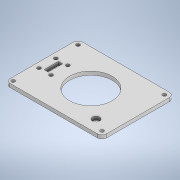
# Autodesk Inventor part: upper_plate_impeller
Saved by Autodesk Inventor 2020 (Build 240168000, 168)
## iProperties
Created: 2023-05-24
Part Number: upper_plate_impeller
Material: Типовые
Document SubType Name: Modeling
Designer: Администратор
Density: 1 g/cm^3
Appearance: По умолчанию
Author: Администратор
Autodesk Inventor part; units mm, degrees
ref_plane "YZ Plane" through (0, 0, 0) normal (1, 0, 0) x (0, 1, 0)
ref_plane "XZ Plane" through (0, 0, 0) normal (0, 1, 0) x (-1, 0, 0)
ref_plane "XY Plane" through (0, 0, 0) normal (0, 0, 1) x (1, 0, 0)
sketch "Эскиз1" plane through (0, 0, 0) normal (0, 1, 0) x (-1, 0, 0)
  line L0 (37, 30) -> (-36, 30)
  line L1 (-40, 26) -> (-40, -26)
  line L2 (-36, -30) -> (36, -30)
  line L3 (40, -26) -> (40, 27)
  line L4 (40, 30) -> (-40, -30) construction
  line L5 (-40, 30) -> (40, -30) construction
  arc A0 (36, -30) -> (40, -26) centre (36, -26) ccw
  arc A1 (40, 27) -> (37, 30) centre (37, 27) ccw
  arc A2 (-40, -26) -> (-36, -30) centre (-36, -26) ccw
  arc A3 (-36, 30) -> (-40, 26) centre (-36, 26) ccw
  circle A4 centre (36, -26) radius 1.5
  circle A5 centre (-36, -26) radius 1.5
  circle A6 centre (-36, 26) radius 1.5
  circle A7 centre (37, 27) radius 1.5
  circle A8 centre (-0.75, 0) radius 17.75
  circle A9 centre (-25, 20) radius 3
  line L6 (40, 0) -> (-40, 0) construction
  circle A10 centre (35.5, -7) radius 1.5
  circle A11 centre (25.5, -7) radius 1.5
  circle A12 centre (35.5, 7) radius 1.5
  circle A13 centre (25.5, 7) radius 1.5
  line L7 (40, 0) -> (23, 0) construction
  line L8 (35.5, -7) -> (25.5, 7) construction
  line L9 (39, -10.5) -> (22, -10.5) construction
  line L10 (22, -10.5) -> (22, 10.5) construction
  line L11 (22, 10.5) -> (39, 10.5) construction
  line L12 (39, 10.5) -> (39, -10.5) construction
  line L13 (32.25, 6) -> (28.75, 6)
  line L14 (28.75, 6) -> (28.75, -6)
  line L15 (28.75, -6) -> (32.25, -6)
  line L16 (32.25, -6) -> (32.25, 6)
  point P0 (0, 0)
  point P1 (30.5, 0)
  dimension "d0" = 80
  dimension "d1" = 60
  dimension "d2" = 4
  dimension "d3" = 3
  dimension "d4" = 4
  dimension "d5" = 3
  dimension "d6" = 3
  dimension "d7" = 3
  dimension "d8" = 3
  dimension "d9" = 35.5
  dimension "d10" = 40.75
  dimension "d13" = 6
  dimension "d14" = 10
  dimension "d15" = 15
  dimension "d16" = 3
  dimension "d17" = 7
  dimension "d18" = 4.5
  dimension "d19" = 3
  dimension "d20" = 10
  dimension "d22" = 17
  dimension "d23" = 21
  dimension "d24" = 3.5
  dimension "d25" = 12
  constraints: 34 end point, 14 centre point, 10 point on line, 8 point on circle, 8 tangent, 6 parallel, 4 coincident, 4 midpoint, 3 horizontal, 3 perpendicular, 2 symmetric about line, 1 equal radius, 2 other
  measures "d0" distance of L5.end L4.end
  measures "d1" distance of L4.end L5.start
  measures "d2" radius of A0
  measures "d3" radius of A1
  measures "d4" radius of A2
  measures "d5" diameter of A4
  measures "d6" diameter of A5
  measures "d7" diameter of A6
  measures "d8" diameter of A7
  measures "d9" diameter of A8
  measures "d10" distance from line of L3 A8.centre
  measures "d13" diameter of A9
  measures "d14" distance from line of L0 A9.centre
  measures "d15" distance from line of L1 A9.centre
  measures "d16" diameter of A10
  measures "d17" distance from line of L6 L8.start
  measures "d18" distance from line of L3 L8.start
  measures "d19" diameter of A11
  measures "d20" distance of A11.centre L8.start
  measures "d22" distance of L10.end L11.end
  measures "d23" distance of L9.end L10.end
  measures "d24" distance of L15.end L14.end
  measures "d25" distance of L14.end L13.end
extrude "Выдавливание1" add sketch "Эскиз1" along normal blind 3
